wall_holder_v1 (Autodesk Fusion 360 design; units mm, degrees)
Autodesk Fusion 360 part; units mm, degrees
sketch "Esquisse1" plane through (0, 0, 0) normal (0, 0, 1) x (1, 0, 0)
  circle A0 centre (0, 0) radius 2.5
  circle A1 centre (0, 0) radius 6.5
  line L0 (0, 6.5) -> (11.5, 6.5)
  line L1 (11.5, 6.5) -> (11.5, -6.5)
  line L2 (11.5, -6.5) -> (0, -6.5)
  line L3 (0, -6.5) -> (0, 6.5) construction
  dimension "d1" = 5
  dimension "d2" = 4
  dimension "d3" = 13
  dimension "d4" = 11.5
  constraint coincident A0.centre A1.centre
  constraint horizontal L0
  constraint vertical L1
  constraint horizontal L2
  constraint vertical L3
  constraint coincident A1 L0.start
  constraint midpoint A0.centre L3
  measures "d1" diameter of A0
  measures "d3" distance of L0.start L2.end
  measures "d4" distance of L0.start L0.end
extrude "Extrusion1" add sketch "Esquisse1" along normal blind 8 makes body 1
sketch "Esquisse3" plane through (0, -6.5, 0) normal (0, -1, 0) x (1, 0, 0)
  line L0 (0, 0) -> (11.5, 0)
  line L1 (11.5, 0) -> (11.5, 8)
  line L2 (11.5, 8) -> (0, 8)
  line L3 (0, 8) -> (0, 0)
  circle A0 centre (7.5, 4) radius 4
  dimension "d14" = 8
  constraint tangent L2 A0
  constraint tangent L1 A0
  measures "d14" diameter of A0
pattern_circular "Réseau C2" count 2 over 90 about axis through (7.5, -6.5, 4) along (0, -1, 0) of bodies 1 makes body 2
sketch "Esquisse2" plane through (0, -6.5, 0) normal (0, -1, 0) x (1, 0, 0)
  line L0 (0, 0) -> (11.5, 0)
  line L1 (11.5, 0) -> (11.5, 8)
  line L2 (11.5, 8) -> (0, 8)
  line L3 (0, 8) -> (0, 0)
  circle A0 centre (7.5, 4) radius 4
  circle A1 centre (7.5, 4) radius 2.5
  line L4 (0, 0) -> (-6.5, 0)
  line L5 (0, 0) -> (0, 8)
  line L6 (0, 8) -> (-6.5, 8)
  line L7 (0, 8) -> (0, 0)
  line L8 (-6.5, 8) -> (-6.5, 0)
  line L9 (7.5, 4) -> (11.5, 8) construction
  line L10 (7.5, 4) -> (7.6746, 8)
  line L11 (7.5, 4) -> (11.5, 4.1746)
  line L12 (7.5, 4) -> (0, 4) construction
  line L13 (7.5, 8) -> (-6.5, 8)
  line L14 (-6.5, 8) -> (-6.5, 2)
  line L15 (7.5, 2) -> (7.5, 8) construction
  line L16 (11.5, -3.5) -> (11.5, -10)
  line L17 (11.5, -3.5) -> (3.5, -3.5)
  line L18 (3.5, -3.5) -> (3.5, -10)
  line L19 (3.5, -3.5) -> (11.5, -3.5)
  line L20 (11.5, -3.5) -> (11.5, 8)
  line L21 (11.5, 8) -> (3.5, 8)
  line L22 (3.5, 8) -> (3.5, -3.5)
  line L23 (3.5, -3.5) -> (11.5, -3.5)
  line L24 (-6.5, 2) -> (3.5, 2)
  line L25 (3.5, -10) -> (11.5, -10)
  line L26 (11.5, 4.1746) -> (11.5, -10)
  line L27 (5.5, -10) -> (5.5, 0.5359)
  line L28 (3.5, 2) -> (4.0359, 2)
  dimension "d7" = 8
  dimension "d8" = 5
  dimension "d21" = 85
  dimension "d22" = 6
  dimension "d26" = 6
  constraint tangent L2 A0
  constraint tangent L1 A0
  constraint concentric A0 A1
  constraint coincident A0.centre A1.centre
  constraint coincident L6.end L8.start
  constraint coincident L4.end L8.end
  constraint coincident L1.end L2.start
  constraint coincident L2 L10.end
  constraint coincident L1 L11.end
  constraint symmetric L9 L10 L11
  constraint midpoint L7 L12.end
  constraint horizontal L13
  constraint vertical L14
  constraint horizontal L24
  constraint vertical L15
  constraint coincident L8 L14.end
  constraint coincident A0 L13.start
  constraint collinear L6 L13
  constraint coincident L16.end L25.end
  constraint perpendicular L16 L25
  constraint coincident L25 L27.start
  constraint coincident A0 L27.end
  constraint perpendicular L0 L27
  constraint coincident A0 L28.end
  constraint perpendicular L22 L28
  measures "d7" diameter of A0
  measures "d8" diameter of A1
  measures "d21" angle of L10 L11
  measures "d22" distance of L13 L24
  measures "d26" distance of L26 L27
extrude "Extrusion4" cut sketch "Esquisse2" against normal through all contours L0 L3 L5 L7 L22 L24 | L3 L4 L5 L7 L8 L24 | L0 A0 L22 L27 L28 | L0 L17 L19 L22 L23 L27 | L17 L18 L19 L23 L25 L27 | L1 L2 A0 L10 L11 L20 L21 | A0 A1 L10 L11 | A1 L10 L11 | A1 L10 L11 picked at (10.9589, 4.4716) bodies 1 2
equation "d3 = d1 + 2 * d2"
equation "d4 = d3 / 2 + 5 mm"
